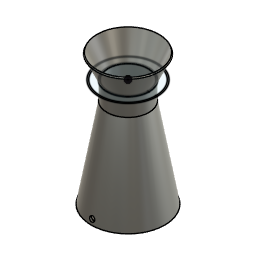
熔岩灯底座 (Autodesk Fusion 360 design; units mm, degrees)
Autodesk Fusion 360 part; units mm, degrees
sketch "草图1" plane through (0, 0, 0) normal (0, 1, 0) x (1, 0, 0)
  circle A0 centre (0, 0) radius 46.5
  circle A1 centre (0, 0) radius 48.5
  circle A2 centre (0, 0) radius 33
  circle A3 centre (0, 0) radius 35
  dimension "d1" = 93
  dimension "d2" = 97
  dimension "d5" = 66
  dimension "d6" = 70
  constraint coincident A0.centre A1.centre
  constraint concentric A0 A2
  measures "d1" diameter of A0
  measures "d2" diameter of A1
  measures "d5" diameter of A2
  measures "d6" diameter of A3
extrude "拉伸2" add sketch "草图1" along normal blind 40 draft 25 contours A3
extrude "拉伸3" cut sketch "草图1" along normal blind 40 draft 25 contours A2
fillet "圆角1" radius 1.5 1 edges at (-50.0215, 40, -19.4015)
extrude "拉伸4" add sketch "草图1" against normal blind 30 contours A3
sketch "草图2" plane through (0, -30, 0) normal (0, -1, 0) x (1, 0, 0)
  circle A0 centre (0, 0) radius 33
  circle A1 centre (0, 0) radius 35
sketch "草图3" plane through (0, -30, 0) normal (0, -1, 0) x (1, 0, 0)
extrude "拉伸5" add sketch "草图2" along normal blind 140 draft 10
delete_face "删除面1" 1 faces at (-19.1093, -43.3333, -23.9623)
extrude "拉伸6" cut sketch "草图2" along normal blind 140 draft 10 contours A0
sketch "草图4" plane through (0, -170, 0) normal (0, -1, 0) x (1, 0, 0)
  circle A0 centre (0, 0) radius 57.6858
  circle A1 centre (0, 0) radius 59.6858
  line L0 (0, 0) -> (9.3, 0)
  line L1 (0, 0) -> (-9.3, 0)
  circle A2 centre (-9.3, 0) radius 3
  circle A3 centre (9.3, 0) radius 3
  dimension "d25" = 9.3
  dimension "d26" = 9.3
  dimension "d27" = 6
  dimension "d28" = 6
  constraint coincident A0.centre A1.centre
  constraint horizontal L0
  constraint parallel L0 L1
  constraint coincident L1.end A2.centre
  constraint coincident L0.end A3.centre
  measures "d25" distance of A0.centre L0.end
  measures "d26" distance of A0.centre L1.end
  measures "d27" diameter of A2
  measures "d28" diameter of A3
extrude "拉伸7" add sketch "草图4" along normal blind 10 draft 10 contours A1
sketch "草图5" plane through (0, -180, 0) normal (0, -1, 0) x (1, 0, 0)
  circle A0 centre (0, 0) radius 55.9225
  circle A1 centre (0, 0) radius 61.449
extrude "拉伸8" add sketch "草图5" against normal blind 2 draft 10 contours A0
extrude "拉伸9" add sketch "草图4" against normal blind 2 contours A0 | A2 | A3
extrude "拉伸10" add sketch "草图4" against normal blind 6 draft -12 contours A2
extrude "拉伸11" add sketch "草图4" against normal blind 6 draft -12 contours A3
hole "孔1" at (0, -171.8844, 60.018) direction (0, -0.173648, -0.984808) diameter 8.526 depth 4 tip angle 180
